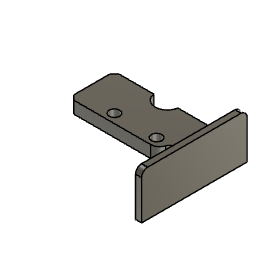
protection tube chauffe v8 (Autodesk Fusion 360 design; units mm, degrees)
Autodesk Fusion 360 part; units mm, degrees
sketch "Esquisse1" plane through (0, 0, 0) normal (0, 0, 1) x (1, 0, 0)
  line L0 (21, -7.5) -> (-21, -7.5)
  line L1 (-21, -7.5) -> (-21, 7.5)
  line L2 (21, 7.5) -> (21, -7.5)
  line L3 (21, -7.5) -> (-21, 7.5) construction
  line L4 (-21, -7.5) -> (21, 7.5) construction
  circle A0 centre (5, -4.5) radius 1.75
  circle A1 centre (-9, -4.5) radius 1.75
  line L5 (-9, -4.5) -> (5, -4.5) construction
  line L6 (-9, -4.5) -> (-9, -7.5) construction
  line L7 (-9, -4.5) -> (-21, -4.5) construction
  line L8 (5, -4.5) -> (21, -4.5) construction
  line L9 (-21, 7.5) -> (21, 7.5)
  line L10 (-21, 7.5) -> (-4, 7.5)
  line L11 (-4, 9) -> (-4, 5.805) construction
  dimension "d1" = 42
  dimension "d2" = 15
  dimension "d3" = 3.5
  dimension "d4" = 3.5
  dimension "d6" = 3
  dimension "d42" = 12
  dimension "d43" = 14
  dimension "d44" = 16
  dimension "d64" = 17
  constraint horizontal L0
  constraint perpendicular L0 L1
  constraint parallel L1 L2
  constraint coincident L3 origin
  constraint coincident L4 origin
  constraint coincident A1.centre L5.start
  constraint coincident A0.centre L5.end
  constraint horizontal L5
  constraint coincident L0 L6.end
  constraint perpendicular L0 L6
  constraint coincident L1 L7.end
  constraint perpendicular L1 L7
  constraint coincident L2 L8.end
  constraint perpendicular L2 L8
  constraint perpendicular L2 L9
  constraint perpendicular L1 L10
  constraint perpendicular L9 L11
  measures "d1" distance of L1.end L2.start
  measures "d2" distance of L0.end L1.end
  measures "d3" diameter of A0
  measures "d4" diameter of A1
  measures "d6" distance of A1.centre L6.end
  measures "d42" distance of A1.centre L7.end
  measures "d43" distance of A1.centre A0.centre
  measures "d44" distance of A0.centre L8.end
  measures "d64" distance of L1.end L10.end
extrude "Extrusion1" add sketch "Esquisse1" along normal blind 4
sketch "Esquisse6" plane through (0, 0, 0) normal (0, 0, 1) x (1, 0, 0)
  line L0 (21, 7.5) -> (23, 7.5)
  line L1 (23, 7.5) -> (23, -27.5)
  line L2 (23, -27.5) -> (21, -27.5)
  line L3 (21, -27.5) -> (21, 7.5)
  dimension "d45" = 2
  dimension "d46" = 35
  constraint horizontal L0
  constraint vertical L1
  constraint horizontal L2
  constraint vertical L3
  measures "d45" distance of L0.start L0.end
  measures "d46" distance of L0.start L2.end
extrude "Extrusion6" add sketch "Esquisse6" along normal blind 15
sketch "Esquisse7" plane through (0, 0, 4) normal (0, 0, 1) x (-1, 0, 0)
  circle A0 centre (-5, 4.5) radius 1.75
  circle A1 centre (9, 4.5) radius 1.75
  line L0 (21, -7.5) -> (21, 7.5)
  line L1 (21, 7.5) -> (-21, 7.5)
  line L2 (-21, 7.5) -> (-21, -7.5)
  line L3 (-21, -7.5) -> (21, -7.5)
  line L4 (-21, 4.0051) -> (-21, 7.5)
  line L5 (-21, 7.5) -> (-5, 7.5)
  line L6 (-8.9589, 4.0051) -> (-21, 4.0051)
  arc A2 (-6, 7.5) -> (-8.9589, 4.0051) centre (-6, 4.5) ccw
  dimension "d70" = 6
  constraint vertical L4
  constraint horizontal L5
  constraint coincident L1.end L2.start
  constraint horizontal L6
  measures "d70" diameter of A2
extrude "Extrusion7" cut sketch "Esquisse7" against normal blind 4 contours L1 L2 L4 L5 L6 A2
chamfer "Chanfrein3" distance 1.5 angle 45 1 edges at (-21, -7.5, 2)
fillet "Congé10" radius 2 1 edges at (21, 1.7475, 4)
fillet "Congé11" radius 2 tangency weight 1.82215 1 edges at (21, -4.0051, 3)
fillet "Congé12" radius 2 tangency weight 0.66524 1 edges at (22, 7.5, 15)
fillet "Congé13" radius 2 1 edges at (22, -27.5, 15)
hole "Perçage1" at (-3.9685, 7.9961, 4) direction (0, 0, -1) diameter 8 end through all
chamfer "Chanfrein5" distance 1.5 angle 45 1 edges at (-21, 7.5, 2)
fillet "Congé14" radius 2 1 edges at (8.9589, -4.0051, 2)
